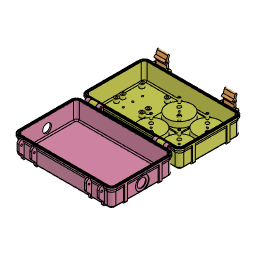
Rugged Relay Box Parametric_Microchallenge 03_MDEF v3 (Autodesk Fusion 360 design; units mm, degrees)
Autodesk Fusion 360 part; units mm, degrees
note: some values were not read from the file. Set by a fixed rule: which face or edge a step refers to.
(part 1 of 2)
sketch "Sketch1" plane through (0, 0, 0) normal (0, 1, 0) x (1, 0, 0) in component "Box"
  line L0 (45, -78) -> (-45, -78)
  line L1 (-48, -75) -> (-48, 75)
  line L2 (-45, 78) -> (45, 78)
  line L3 (48, 75) -> (48, -75)
  line L4 (48, -78) -> (-48, 78) construction
  line L5 (-48, -78) -> (48, 78) construction
  arc A0 (-45, 78) -> (-48, 75) centre (-45, 75) ccw
  arc A1 (48, 75) -> (45, 78) centre (45, 75) ccw
  arc A2 (45, -78) -> (48, -75) centre (45, -75) ccw
  arc A3 (-48, -75) -> (-45, -78) centre (-45, -75) ccw
  dimension "d6" = 156
  dimension "d7" = 96
  dimension "d9" = 3
  constraint horizontal L0
  constraint perpendicular L0 L1
  constraint parallel L0 L2
  constraint parallel L1 L3
  constraint coincident L4 origin
  constraint coincident L5 origin
  constraint coincident L4.end L2
  constraint coincident L4.end L1
  constraint tangent L2 A0
  constraint tangent L1 A0
  constraint coincident L5.end L2
  constraint coincident L5.end L3
  constraint tangent L2 A1
  constraint tangent L3 A1
  constraint coincident L4.start L3
  constraint coincident L4.start L0
  constraint tangent L3 A2
  constraint tangent L0 A2
  constraint coincident L5.start L0
  constraint coincident L5.start L1
  constraint tangent L0 A3
  constraint tangent L1 A3
  constraint equal A0 A1
  constraint equal A0 A3
  constraint equal A2 A3
  measures "d6" distance of L0 L2
  measures "d7" distance of L1 L3
  measures "d9" radius of A1
sketch "Sketch2" plane through (0, 0, 0) normal (0, 0, 1) x (1, 0, 0) in component "Box"
  line L0 (0, 0) -> (48, 0)
  line L1 (48, 0) -> (48, 2.4)
  line L2 (50, 4.4) -> (50, 32.4)
  line L3 (50, 32.4) -> (51.23, 32.4)
  line L4 (51.23, 32.4) -> (51.23, 30.4)
  line L5 (51.23, 30.4) -> (53.03, 30.4)
  line L6 (53.03, 30.4) -> (53.03, 32.4)
  line L7 (53.03, 32.4) -> (54.26, 32.4)
  line L8 (54.26, 32.4) -> (54.26, 29.4)
  line L9 (58.1865, 0) -> (48, 0)
  line L10 (54.26, 29.4) -> (52.4, 29.4)
  line L11 (52.4, 29.4) -> (52.4, 25)
  line L12 (52.4, 25) -> (52.4, 3.4059)
  line L13 (52.4, 25) -> (54.26, 29.4)
  line L14 (50, 4.4) -> (48, 2.4)
  line L15 (48.9941, 0) -> (52.4, 3.4059)
  line L16 (58.1865, 0) -> (61.26, 3.0735)
  line L17 (54.26, 32.4) -> (56.26, 32.4)
  line L18 (61.26, 27.4) -> (61.26, 3.0735)
  arc A0 (61.26, 27.4) -> (56.26, 32.4) centre (56.26, 27.4) ccw
  circle A1 centre (56.76, 24.4) radius 1.7
  line L19 (0, 0) -> (0, 60)
  line L20 (-61.26, 27.4) -> (-61.26, 3.0735)
  line L21 (-51.23, 32.4) -> (-51.23, 30.4)
  line L22 (-52.4, 25) -> (-54.26, 29.4)
  line L23 (-50, 4.4) -> (-50, 32.4)
  line L24 (-48, 0) -> (-48, 2.4)
  line L25 (-51.23, 30.4) -> (-53.03, 30.4)
  line L26 (-48.9941, 0) -> (-52.4, 3.4059)
  line L27 (-52.4, 25) -> (-52.4, 3.4059)
  line L28 (-50, 4.4) -> (-48, 2.4)
  line L29 (-54.26, 32.4) -> (-54.26, 29.4)
  line L30 (-58.1865, 0) -> (-61.26, 3.0735)
  line L31 (-52.4, 29.4) -> (-52.4, 25)
  line L32 (-53.03, 32.4) -> (-54.26, 32.4)
  line L33 (-53.03, 30.4) -> (-53.03, 32.4)
  line L34 (-58.1865, 0) -> (-48, 0)
  line L35 (-54.26, 29.4) -> (-52.4, 29.4)
  line L36 (-50, 32.4) -> (-51.23, 32.4)
  line L37 (52.4, 29.4) -> (50, 29.4)
  line L38 (-52.4, 29.4) -> (-50, 29.4)
  circle A2 centre (-57.86, 32.4) radius 1.7
  circle A3 centre (-57.86, 32.4) radius 3.4
  line L39 (-61.26, 32.4) -> (-61.26, 27.4)
  line L40 (-54.26, 32.4) -> (-54.46, 32.4)
  line L41 (-60.2642, 29.9958) -> (-50, 19.7317)
  line L42 (-60.2642, 29.9958) -> (-39.091, 29.9958) construction
  line L43 (-57.86, 32.4) -> (-54.26, 32.4)
  line L44 (51.6245, 0) -> (54.26, 2.6355)
  line L45 (54.26, 2.6355) -> (54.26, 8.4)
  line L46 (54.26, 8.4) -> (61.26, 15.4)
  line L47 (-51.6245, 0) -> (-54.26, 2.6355)
  line L48 (-54.26, 2.6355) -> (-54.26, 20.4)
  line L49 (-54.26, 20.4) -> (-61.26, 27.4)
  point P0 (61.26, 32.4)
  point P1 (-61.26, 32.4)
  dimension "d12" = 48
  dimension "d13" = 2.4
  dimension "d15" = 1.23
  dimension "d16" = 2
  dimension "d17" = 1.8
  dimension "d18" = 2
  dimension "d20" = 3
  dimension "d23" = 4.4
  dimension "d26" = 2.4
  dimension "d27" = 2
  dimension "d28" = 2
  dimension "d29" = 32.4
  dimension "d30" = 6.5
  dimension "d61" = 7
  dimension "d62" = 5
  dimension "d63" = 3.4
  dimension "d64" = 8
  dimension "d65" = 4.5
  dimension "d129" = 1.23
  dimension "d131" = 2.4
  dimension "d137" = 3.4
  dimension "d138" = 3.6
  dimension "d139" = 6.8
  dimension "d140" = 45
  dimension "d111" = 1.86
  dimension "d113" = 1.86
  dimension "d114" = 17
  dimension "d123" = 5
  constraint coincident L0.start L19.start
  constraint horizontal L0
  constraint perpendicular L0 L1
  constraint perpendicular L2 L3
  constraint perpendicular L3 L4
  constraint perpendicular L4 L5
  constraint perpendicular L5 L6
  constraint perpendicular L6 L7
  constraint perpendicular L7 L8
  constraint perpendicular L1 L9
  constraint perpendicular L8 L10
  constraint perpendicular L10 L11
  constraint perpendicular L9 L12
  constraint coincident L9 L15.start
  constraint vertical L2
  constraint perpendicular L8 L17
  constraint perpendicular L7 L18
  constraint coincident P0 L17
  constraint coincident P0 L18
  constraint tangent L17 A0
  constraint tangent L18 A0
  constraint perpendicular L0 L19
  constraint symmetric L0.end L19 L24.start
  constraint symmetric L1.end L19 L24.end
  constraint symmetric L2.end L19 L23.end
  constraint symmetric L3.end L19 L21.start
  constraint symmetric L4.end L19 L21.end
  constraint symmetric L5.end L19 L25.end
  constraint symmetric L6.end L19 L32.start
  constraint symmetric L7.end L19 L29.start
  constraint symmetric L8.end L19 L22.end
  constraint symmetric L10.end L19 L31.start
  constraint symmetric L11.end L19 L22.start
  constraint symmetric L2.start L19 L23.start
  constraint symmetric L15.start L19 L26.start
  constraint symmetric L12.end L19 L26.end
  constraint symmetric L9.start L19 L30.start
  constraint symmetric P0 L19 P1
  constraint symmetric L16.end L19 L20.end
  constraint symmetric L18.start L19 L20.start
  constraint coincident L2 L37.end
  constraint perpendicular L2 L37
  constraint coincident L23 L38.end
  constraint perpendicular L23 L38
  constraint concentric A2 A3
  constraint coincident P1 L39.start
  constraint coincident A3 L40.end
  constraint horizontal L42
  constraint coincident A3 L41.start
  constraint tangent A3 L41
  constraint coincident L23 L41.end
  constraint coincident A2.centre A3.centre
  constraint perpendicular L29 L43
  constraint horizontal L40
  constraint coincident L9 L44.start
  constraint perpendicular L9 L45
  constraint coincident L18 L46.end
  constraint collinear L8 L45
  constraint parallel L15 L44
  constraint symmetric L19 L44.start L47.start
  constraint symmetric L19 L44.end L47.end
  constraint parallel L44 L46
  constraint parallel L27 L48
  constraint coincident L20 L39.end
  constraint parallel L47 L49
  measures "d12" distance of L0.start L0.end
  measures "d13" distance of L0.end L1.end
  measures "d15" distance of L2.end L3.end
  measures "d16" distance of L3.end L4.end
  measures "d17" distance of L4.end L5.end
  measures "d18" distance of L5.end L6.end
  measures "d20" distance of L7.end L8.end
  measures "d23" distance of L10.end L11.end
  measures "d26" distance of L14 L15
  measures "d27" vertical distance of L1.end L2.start
  measures "d28" horizontal distance of L1.end L2.start
  measures "d29" distance of L0.end L7
  measures "d30" distance of L15 L16
  measures "d61" distance of L7.end P0
  measures "d62" radius of A0
  measures "d63" diameter of A1
  measures "d64" distance of L17 A1.centre
  measures "d65" distance of L18 A1.centre
  measures "d129" distance of L6 L8
  measures "d131" distance of L2 L12
  measures "d137" diameter of A2
  measures "d138" distance of L29.start A2.centre
  measures "d139" diameter of A3
  measures "d140" angle of L41 L42
  measures "d111" distance of L15 L44
  measures "d113" distance of L8 L11
  measures "d114" distance of L17 L46.end
  measures "d123" distance of L43 L20.start
extrude "Extrude1" add sketch "Sketch1" along normal blind 2.4 makes body 1 in component "Box"
sweep "Sweep1" add profiles "Sketch2" path "Sketch1" along A2 L0 A3 L1 A0 L2 A1 L3 section 1 contours L1 L2 L9 L11 L12 L14 L15 L37 | L2 L3 L4 L5 L6 L7 L8 L10 L37 | L10 L11 L13 bodies 1 in component "Box"
ref_plane "WorkPlane2" through (-32, 0, 0) normal (1, 0, 0) x (0, 1, 0) in component "Box"
sketch "Sketch4" plane through (-32, 0, 0) normal (1, 0, 0) x (0, 0, -1) in component "Box"
  line L0 (0, 0) -> (-78, 0)
  line L1 (-78, 0) -> (-78, 2.4)
  line L2 (-78, 2.4) -> (-80, 2.4)
  line L3 (-80, 2.4) -> (-80, 4.4)
  line L4 (-80, 4.4) -> (-78, 2.4)
  line L5 (-80, 2.4) -> (-80, 5)
  line L6 (-80, 2.4) -> (-80, 29.4)
  line L7 (-80, 29.4) -> (-84.26, 29.4)
  line L8 (-84.26, 29.4) -> (-84.26, 2.6355)
  line L9 (-81.6245, 0) -> (-78, 0)
  line L10 (-81.6245, 0) -> (-84.26, 2.6355)
  line L11 (0, 0) -> (0, 70)
  line L12 (81.6245, 0) -> (84.26, 2.6355)
  line L13 (81.6245, 0) -> (78, 0)
  line L14 (80, 2.4) -> (80, 5)
  line L15 (80, 2.4) -> (80, 29.4)
  line L16 (80, 4.4) -> (78, 2.4)
  line L17 (80, 2.4) -> (80, 4.4)
  line L18 (80, 29.4) -> (84.26, 29.4)
  line L19 (84.26, 29.4) -> (84.26, 2.6355)
  line L20 (78, 0) -> (78, 2.4)
  line L21 (78, 2.4) -> (80, 2.4)
  dimension "d47" = 78
  dimension "d48" = 2.4
  dimension "d49" = 2
  dimension "d50" = 2
  dimension "d52" = 4.26
  dimension "d53" = 4.26
  dimension "d56" = 29.4
  constraint coincident L0.start L11.start
  constraint horizontal L0
  constraint perpendicular L0 L1
  constraint perpendicular L1 L2
  constraint perpendicular L2 L3
  constraint coincident L3 L5.end
  constraint perpendicular L2 L6
  constraint perpendicular L6 L7
  constraint perpendicular L7 L8
  constraint perpendicular L1 L9
  constraint perpendicular L0 L11
  constraint symmetric L0.end L11 L13.end
  constraint symmetric L1.end L11 L16.end
  constraint symmetric L2.end L11 L14.start
  constraint symmetric L3.end L11 L16.start
  constraint symmetric L5.end L11 L14.end
  constraint symmetric L6.end L11 L15.end
  constraint symmetric L7.end L11 L18.end
  constraint symmetric L8.end L11 L12.end
  constraint symmetric L9.start L11 L12.start
  measures "d47" distance of L0.start L0.end
  measures "d48" distance of L0.end L1.end
  measures "d49" distance of L1.end L2.end
  measures "d50" distance of L2.end L3.end
  measures "d52" distance of L6.end L7.end
  measures "d53" distance of L4 L10
  measures "d56" distance of L7 L9
extrude "Extrude2" add sketch "Sketch4" along normal blind 5 bodies 1 in component "Box"
ref_plane "WorkPlane3" through (32, 0, 0) normal (1, 0, 0) x (0, 1, 0) in component "Box"
sketch "Sketch5" plane through (32, 0, 0) normal (1, 0, 0) x (0, 0, -1) in component "Box"
  line L0 (-80, 2.4) -> (-80, 29.4)
  line L1 (-80, 4.4) -> (-78, 2.4)
  line L2 (-78, 2.4) -> (-80, 2.4)
  line L3 (-78, 0) -> (-78, 2.4)
  line L4 (-81.6245, 0) -> (-78, 0)
  line L5 (-81.6245, 0) -> (-84.26, 2.6355)
  line L6 (-84.26, 29.4) -> (-84.26, 2.6355)
  line L7 (-80, 29.4) -> (-84.26, 29.4)
  line L8 (80, 29.4) -> (84.26, 29.4)
  line L9 (84.26, 29.4) -> (84.26, 2.6355)
  line L10 (80, 2.4) -> (80, 29.4)
  line L11 (80, 4.4) -> (78, 2.4)
  line L12 (78, 2.4) -> (80, 2.4)
  line L13 (81.6245, 0) -> (84.26, 2.6355)
  line L14 (78, 0) -> (78, 2.4)
  line L15 (81.6245, 0) -> (78, 0)
extrude "Extrude3" add sketch "Sketch5" against normal blind 5 bodies 1 in component "Box"
ref_plane "WorkPlane4" through (0, 0, -70) normal (0, 0, 1) x (1, 0, 0) in component "Box"
sketch "Sketch6" plane through (0, 0, -70) normal (0, 0, 1) x (1, 0, 0) in component "Box"
  line L0 (54.26, 32.4) -> (56.26, 32.4)
  line L1 (61.26, 27.4) -> (61.26, 3.0735)
  arc A0 (61.26, 27.4) -> (56.26, 32.4) centre (56.26, 27.4) ccw
  line L2 (58.1865, 0) -> (61.26, 3.0735)
  line L3 (58.1865, 0) -> (48, 0)
  line L4 (48, 0) -> (48, 2.4)
  line L5 (50, 4.4) -> (48, 2.4)
  line L6 (50, 4.4) -> (50, 32.4)
  line L7 (52.4, 29.4) -> (50, 29.4)
  line L8 (54.26, 29.4) -> (52.4, 29.4)
  line L9 (54.26, 32.4) -> (54.26, 29.4)
  line L10 (-50, 4.4) -> (-50, 32.4)
  line L11 (-52.4, 29.4) -> (-50, 29.4)
  line L12 (-54.26, 29.4) -> (-52.4, 29.4)
  line L13 (-54.26, 32.4) -> (-54.26, 29.4)
  line L14 (-61.26, 27.4) -> (-61.26, 3.0735)
  line L15 (-58.1865, 0) -> (-61.26, 3.0735)
  line L16 (-58.1865, 0) -> (-48, 0)
  line L17 (-48, 0) -> (-48, 2.4)
  line L18 (-50, 4.4) -> (-48, 2.4)
  circle A1 centre (56.76, 24.4) radius 1.7
  line L19 (-61.26, 32.4) -> (-61.26, 27.4)
  circle A2 centre (-57.86, 32.4) radius 3.4
  circle A3 centre (-57.86, 32.4) radius 1.7
  line L20 (-54.26, 32.4) -> (-54.46, 32.4)
  line L21 (-60.2642, 29.9958) -> (-50, 19.7317)
  line L22 (54.26, 8.4) -> (61.26, 15.4)
  line L23 (54.26, 2.6355) -> (54.26, 8.4)
  line L24 (51.6245, 0) -> (54.26, 2.6355)
  line L25 (-51.6245, 0) -> (-54.26, 2.6355)
  line L26 (-54.26, 2.6355) -> (-54.26, 20.4)
  line L27 (-54.26, 20.4) -> (-61.26, 27.4)
  point P0 (61.26, 32.4)
  point P1 (56.76, 24.4)
extrude "Extrude10" add sketch "Sketch6" along normal blind 3.2 contours L0 L1 A0 L3 L4 L5 L6 L7 L8 L9 L22 L23 L24 | L10 L16 L17 L18 L19 A2 L21 L25 L26 L27 | L10 L11 L12 L13 A2 L20 L21 | A2 bodies 1 in component "Box"
extrude "Extrude17" add sketch "Sketch6" along normal blind 6.2 contours L10 L11 L12 L13 A2 L20 L21 | A2 bodies 1 in component "Box"
ref_plane "WorkPlane5" through (0, 0, -45) normal (0, 0, 1) x (1, 0, 0) in component "Box"
sketch "Sketch7" plane through (0, 0, -45) normal (0, 0, 1) x (1, 0, 0) in component "Box"
  line L0 (-48, 0) -> (-48, 2.4)
  line L1 (-50, 4.4) -> (-48, 2.4)
  line L2 (-50, 4.4) -> (-50, 32.4)
  line L3 (-52.4, 29.4) -> (-50, 29.4)
  line L4 (-54.26, 29.4) -> (-52.4, 29.4)
  line L5 (-54.26, 32.4) -> (-54.26, 29.4)
  line L6 (-61.26, 27.4) -> (-61.26, 3.0735)
  line L7 (-58.1865, 0) -> (-61.26, 3.0735)
  line L8 (-58.1865, 0) -> (-48, 0)
  line L9 (48, 0) -> (48, 2.4)
  line L10 (50, 4.4) -> (48, 2.4)
  line L11 (50, 4.4) -> (50, 32.4)
  line L12 (52.4, 29.4) -> (50, 29.4)
  line L13 (54.26, 29.4) -> (52.4, 29.4)
  line L14 (54.26, 32.4) -> (54.26, 29.4)
  line L15 (54.26, 32.4) -> (56.26, 32.4)
  arc A0 (61.26, 27.4) -> (56.26, 32.4) centre (56.26, 27.4) ccw
  line L16 (61.26, 27.4) -> (61.26, 3.0735)
  line L17 (58.1865, 0) -> (61.26, 3.0735)
  line L18 (58.1865, 0) -> (48, 0)
  circle A1 centre (56.76, 24.4) radius 1.7 construction
  line L19 (-61.26, 32.4) -> (-61.26, 27.4)
  circle A2 centre (-57.86, 32.4) radius 3.4
  line L20 (-54.26, 32.4) -> (-54.46, 32.4)
  circle A3 centre (-57.86, 32.4) radius 1.7 construction
  line L21 (-60.2642, 29.9958) -> (-50, 19.7317)
  circle A4 centre (56.76, 24.4) radius 1.425
  circle A5 centre (-57.86, 32.4) radius 1.425
  line L22 (-51.6245, 0) -> (-54.26, 2.6355)
  line L23 (54.26, 8.4) -> (61.26, 15.4)
  line L24 (54.26, 2.6355) -> (54.26, 8.4)
  line L25 (51.6245, 0) -> (54.26, 2.6355)
  line L26 (-54.26, 2.6355) -> (-54.26, 20.4)
  line L27 (-54.26, 20.4) -> (-61.26, 27.4)
  dimension "d24" = 2.85
  dimension "d25" = 2.85
  constraint concentric A1 A4
  constraint concentric A2 A5
  measures "d24" diameter of A4
  measures "d25" diameter of A5
extrude "Extrude11" add sketch "Sketch7" against normal blind 3.2 contours L0 L1 L2 L8 L19 A2 L21 L22 L26 L27 | L2 L3 L4 L5 A2 L20 L21 | A2 | L9 L10 L11 L12 L13 L14 L15 A0 L16 L18 L23 L24 L25 bodies 1 in component "Box"
extrude "Extrude18" add sketch "Sketch7" against normal blind 6.2 contours L2 L3 L4 L5 A2 L20 L21 | A2 bodies 1 in component "Box"
ref_plane "WorkPlane6" through (0, 0, 70) normal (0, 0, 1) x (1, 0, 0) in component "Box"
sketch "Sketch8" plane through (0, 0, 70) normal (0, 0, 1) x (1, 0, 0) in component "Box"
  line L0 (-61.26, 27.4) -> (-61.26, 3.0735)
  line L1 (-54.26, 32.4) -> (-54.26, 29.4)
  line L2 (-54.26, 29.4) -> (-52.4, 29.4)
  line L3 (-52.4, 29.4) -> (-50, 29.4)
  line L4 (-50, 4.4) -> (-50, 32.4)
  line L5 (-50, 4.4) -> (-48, 2.4)
  line L6 (-48, 0) -> (-48, 2.4)
  line L7 (-58.1865, 0) -> (-48, 0)
  line L8 (-58.1865, 0) -> (-61.26, 3.0735)
  line L9 (48, 0) -> (48, 2.4)
  line L10 (50, 4.4) -> (48, 2.4)
  line L11 (50, 4.4) -> (50, 32.4)
  line L12 (52.4, 29.4) -> (50, 29.4)
  line L13 (54.26, 29.4) -> (52.4, 29.4)
  line L14 (54.26, 32.4) -> (54.26, 29.4)
  line L15 (54.26, 32.4) -> (56.26, 32.4)
  arc A0 (61.26, 27.4) -> (56.26, 32.4) centre (56.26, 27.4) ccw
  line L16 (61.26, 27.4) -> (61.26, 3.0735)
  line L17 (58.1865, 0) -> (61.26, 3.0735)
  circle A1 centre (56.76, 24.4) radius 1.7
  line L18 (58.1865, 0) -> (48, 0)
  line L19 (-61.26, 32.4) -> (-61.26, 27.4)
  circle A2 centre (-57.86, 32.4) radius 3.4
  circle A3 centre (-57.86, 32.4) radius 1.7
  line L20 (-54.26, 32.4) -> (-54.46, 32.4)
  line L21 (-60.2642, 29.9958) -> (-50, 19.7317)
  line L22 (54.26, 8.4) -> (61.26, 15.4)
  line L23 (54.26, 2.6355) -> (54.26, 8.4)
  line L24 (51.6245, 0) -> (54.26, 2.6355)
  line L25 (-51.6245, 0) -> (-54.26, 2.6355)
  line L26 (-54.26, 2.6355) -> (-54.26, 20.4)
  line L27 (-54.26, 20.4) -> (-61.26, 27.4)
extrude "Extrude12" add sketch "Sketch8" against normal blind 3.2 contours L4 L5 L6 L7 L19 A2 L21 L25 L26 L27 | A2 | L1 L2 L3 L4 A2 L20 L21 | L9 L10 L11 L12 L13 L14 L15 A0 L16 L18 L22 L23 L24 bodies 1 in component "Box"
extrude "Extrude19" add sketch "Sketch8" against normal blind 6.2 contours A2 | L1 L2 L3 L4 A2 L20 L21 bodies 1 in component "Box"
ref_plane "WorkPlane7" through (0, 0, 45) normal (0, 0, 1) x (1, 0, 0) in component "Box"
sketch "Sketch9" plane through (0, 0, 45) normal (0, 0, 1) x (1, 0, 0) in component "Box"
  line L0 (58.1865, 0) -> (61.26, 3.0735)
  line L1 (58.1865, 0) -> (48, 0)
  line L2 (61.26, 27.4) -> (61.26, 3.0735)
  arc A0 (61.26, 27.4) -> (56.26, 32.4) centre (56.26, 27.4) ccw
  line L3 (54.26, 32.4) -> (56.26, 32.4)
  line L4 (54.26, 32.4) -> (54.26, 29.4)
  line L5 (54.26, 29.4) -> (52.4, 29.4)
  line L6 (52.4, 29.4) -> (50, 29.4)
  line L7 (50, 4.4) -> (50, 32.4)
  line L8 (50, 4.4) -> (48, 2.4)
  line L9 (48, 0) -> (48, 2.4)
  line L10 (-48, 0) -> (-48, 2.4)
  line L11 (-50, 4.4) -> (-48, 2.4)
  line L12 (-50, 4.4) -> (-50, 32.4)
  line L13 (-52.4, 29.4) -> (-50, 29.4)
  line L14 (-54.26, 29.4) -> (-52.4, 29.4)
  line L15 (-54.26, 32.4) -> (-54.26, 29.4)
  line L16 (-61.26, 27.4) -> (-61.26, 3.0735)
  line L17 (-58.1865, 0) -> (-61.26, 3.0735)
  line L18 (-58.1865, 0) -> (-48, 0)
  circle A1 centre (56.76, 24.4) radius 1.7 construction
  line L19 (-61.26, 32.4) -> (-61.26, 27.4)
  circle A2 centre (-57.86, 32.4) radius 3.4
  circle A3 centre (-57.86, 32.4) radius 1.7 construction
  line L20 (-54.26, 32.4) -> (-54.46, 32.4)
  line L21 (-60.2642, 29.9958) -> (-50, 19.7317)
  circle A4 centre (56.76, 24.4) radius 1.425
  circle A5 centre (-57.86, 32.4) radius 1.425
  line L22 (54.26, 8.4) -> (61.26, 15.4)
  line L23 (54.26, 2.6355) -> (54.26, 8.4)
  line L24 (51.6245, 0) -> (54.26, 2.6355)
  line L25 (-51.6245, 0) -> (-54.26, 2.6355)
  line L26 (-54.26, 2.6355) -> (-54.26, 20.4)
  line L27 (-54.26, 20.4) -> (-61.26, 27.4)
  point P0 (56.26, 27.4)
  dimension "d39" = 2.85
  dimension "d40" = 2.85
  constraint concentric A1 A4
  constraint concentric A2 A5
  measures "d39" diameter of A4
  measures "d40" diameter of A5
extrude "Extrude13" add sketch "Sketch9" along normal blind 3.2 contours L1 L2 A0 L3 L4 L5 L6 L7 L8 L9 L22 L23 L24 | L10 L11 L12 L18 L19 A2 L21 L25 L26 L27 | L12 L13 L14 L15 A2 L20 L21 | A2 bodies 1 in component "Box"
extrude "Extrude20" add sketch "Sketch9" along normal blind 6.2 contours L12 L13 L14 L15 A2 L20 L21 | A2 bodies 1 in component "Box"
fillet "Fillet2" radius 1 40 edges at (-54.26, 2.6355, 68.4) (-54.26, 20.4, 68.4) (-54.26, 20.4, 46.6) (-54.26, 2.6355, 46.6) (-54.26, 2.6355, -46.6) (-54.26, 20.4, -46.6) (-54.26, 20.4, -68.4) (-54.26, 2.6355, -68.4) (-29.5, 2.6355, 84.26) (29.5, 2.6355, 84.26) (54.26, 2.6355, 68.4) (54.26, 8.4, 68.4) (54.26, 2.6355, 46.6) (54.26, 8.4, 46.6) (54.26, 8.4, -46.6) (54.26, 2.6355, -46.6) (54.26, 2.6355, -68.4) (54.26, 8.4, -68.4) (29.5, 2.6355, -84.26) (-29.5, 2.6355, -84.26) (52.4, 3.4059, 72.5) (50.2326, 3.4059, 80.2326) (38.5, 3.4059, 82.4) (0, 3.4059, 82.4) (-38.5, 3.4059, 82.4) (-50.2326, 3.4059, 80.2326) (-52.4, 3.4059, 72.5) (52.4, 3.4059, 57.5) (52.4, 3.4059, 0) (52.4, 3.4059, -57.5) (38.5, 3.4059, -82.4) (50.2326, 3.4059, -80.2326) (52.4, 3.4059, -72.5) (0, 3.4059, -82.4) (-52.4, 3.4059, -72.5) (-50.2326, 3.4059, -80.2326) (-38.5, 3.4059, -82.4) (-52.4, 3.4059, -57.5) (-52.4, 3.4059, 0) (-52.4, 3.4059, 57.5) 17 faces at (-50.7477, 0, 46.0667) (-50.7477, 0, 68.9333) (-50.7477, 0, -46.0667) (-49.8709, 0, -67.8667) (50.7477, 0, -68.9333) (50.7477, 0, -46.0667) (50.7477, 0, 46.0667) (50.7477, 0, 68.9333) (-48.3314, 0, -22.2667) (30.3333, 0, -79.8709) (-28.6667, 0, -79.8709) (48.3314, 0, 22.2667) (28.6667, 0, 79.8709) (-30.3333, 0, 79.8709) (16, 0, 25) (10.6667, 0, -78.3314) (10.6667, 0, 78.3314) on bodies 1 in component "Box"
fillet "Fillet3" radius 3 8 edges at (61.26, 15.4, 68.4) (61.26, 15.4, 46.6) (61.26, 15.4, -46.6) (61.26, 15.4, -68.4) (-61.26, 27.4, -68.4) (-61.26, 27.4, -46.6) (-61.26, 27.4, 46.6) (-61.26, 27.4, 68.4) on bodies 1 in component "Box"
copy_body "Body->Comp1" bodies 1 removing the originals makes body 2 in component "Box (1)"
sketch "Sketch10" plane through (0, 0, 0) normal (0, 0, 1) x (1, 0, 0) in component "Box"
  circle A0 centre (152.4867, 44.0068) radius 1.6
  circle A1 centre (152.4867, 44.0068) radius 4
  circle A2 centre (152.4867, 60.0068) radius 1.6
  circle A3 centre (152.4867, 60.0068) radius 4
  arc A4 (152.4867, 60.0068) -> (152.4867, 44.0068) centre (171.1154, 52.0068) ccw
  arc A5 (151.0165, 60.6382) -> (151.0165, 43.3755) centre (171.1154, 52.0068) ccw
  arc A6 (153.9568, 59.3755) -> (153.9568, 44.6382) centre (171.1154, 52.0068) ccw
  line L0 (153.4854, 42.7568) -> (156.2863, 42.7568)
  line L1 (152.4867, 44.0068) -> (149.3136, 34.5236)
  circle A7 centre (149.3136, 34.5236) radius 1.6
  line L2 (150.9693, 44.5145) -> (147.7963, 35.0313)
  line L3 (154.004, 43.4992) -> (150.8309, 34.0159)
  line L4 (152.4973, 45.6068) -> (152.8792, 47.9875)
  line L5 (152.4867, 60.0068) -> (152.4867, 44.0068) construction
  dimension "d98" = 3.2
  dimension "d99" = 8
  dimension "d100" = 16
  dimension "d101" = 3.2
  dimension "d102" = 8
  dimension "d105" = 3.2
  dimension "d66" = 10
  dimension "d67" = 161.5
  dimension "d69" = 1.25
  constraint concentric A0 A1
  constraint coincident A0.centre A1.centre
  constraint coincident A2.centre A3.centre
  constraint concentric A2 A3
  constraint coincident A0 L0.start
  constraint coincident A1 L0.end
  constraint coincident L1.end A7.centre
  constraint coincident A0 L4.start
  constraint coincident A6 L4.end
  constraint coincident A1 L4.end
  constraint concentric A4 A6
  constraint concentric A4 A5
  constraint vertical L5
  constraint coincident A2 A6.start
  constraint tangent A2 A6
  constraint tangent A2 A5
  constraint coincident A2 A5.start
  constraint coincident A0 A5.end
  constraint coincident A0 A6.end
  constraint parallel L1 L2
  constraint parallel L1 L3
  constraint coincident A0 L3.start
  constraint coincident A0 L2.start
  constraint tangent A0 L2
  constraint tangent A0 L3
  constraint coincident A7 L2.end
  constraint coincident A7 L3.end
  constraint horizontal L0
  measures "d98" diameter of A0
  measures "d99" diameter of A1
  measures "d100" distance of A0.centre A2.centre
  measures "d101" diameter of A2
  measures "d102" diameter of A3
  measures "d105" diameter of A7
  measures "d66" distance of A0.centre L1.end
  measures "d67" angle of L1 L5
  measures "d69" distance of A0.centre L0
extrude "Extrude15" add sketch "Sketch10" along normal blind 18.2 separate body contours A0 A1 A4 L4 | A1 A3 A4 A6 | A0 A1 L0 L1 L3 | A1 L0 L3 | A0 A1 A4 A5 L2 | A1 A3 A4 A5 | A2 A3 A5 A6 | A2 A3 A4 A6 | A0 A1 A5 L1 L2 | A1 L1 A7 L3 | A1 A5 L2 | A2 A3 A4 A5 | A1 L1 A7 L2 | A7 makes body 3 in component "Box"
copy_body "Body->Comp3" bodies 3 removing the originals makes body 4 in component "Box Latch"
sketch "Sketch1 (2)" plane through (0, 0, 0) normal (0, 1, 0) x (1, 0, 0) in component "Lid"
  line L0 (45, -78) -> (-45, -78)
  line L1 (-48, -75) -> (-48, 75)
  line L2 (-45, 78) -> (45, 78)
  line L3 (48, 75) -> (48, -75)
  line L4 (48, -78) -> (-48, 78) construction
  line L5 (-48, -78) -> (48, 78) construction
  arc A0 (-45, 78) -> (-48, 75) centre (-45, 75) ccw
  arc A1 (48, 75) -> (45, 78) centre (45, 75) ccw
  arc A2 (45, -78) -> (48, -75) centre (45, -75) ccw
  arc A3 (-48, -75) -> (-45, -78) centre (-45, -75) ccw
  dimension "d6_1" = 156
  dimension "d7_1" = 96
  dimension "d9_1" = 3
  constraint horizontal L0
  constraint perpendicular L0 L1
  constraint parallel L0 L2
  constraint parallel L1 L3
  constraint coincident L4 origin
  constraint coincident L5 origin
  constraint coincident L4.end L2
  constraint coincident L4.end L1
  constraint tangent L2 A0
  constraint tangent L1 A0
  constraint coincident L5.end L2
  constraint coincident L5.end L3
  constraint tangent L2 A1
  constraint tangent L3 A1
  constraint coincident L4.start L3
  constraint coincident L4.start L0
  constraint tangent L3 A2
  constraint tangent L0 A2
  constraint coincident L5.start L0
  constraint coincident L5.start L1
  constraint tangent L0 A3
  constraint tangent L1 A3
  constraint equal A0 A1
  constraint equal A0 A3
  constraint equal A2 A3
  measures "d6_1" distance of L0 L2
  measures "d7_1" distance of L1 L3
  measures "d9_1" radius of A1
sketch "Sketch2 (2)" plane through (0, 0, 0) normal (0, 0, 1) x (1, 0, 0) in component "Lid"
  line L0 (0, 0) -> (48, 0)
  line L1 (48, 0) -> (48, 2.4)
  line L2 (50, 4.4) -> (50, 32.4)
  line L3 (50, 32.4) -> (51.23, 32.4)
  line L4 (51.23, 32.4) -> (51.23, 30.4)
  line L5 (51.23, 30.4) -> (53.03, 30.4)
  line L6 (53.03, 30.4) -> (53.03, 32.4)
  line L7 (53.03, 32.4) -> (54.26, 32.4)
  line L8 (54.26, 32.4) -> (54.26, 29.4)
  line L9 (58.1865, 0) -> (48, 0)
  line L10 (54.26, 29.4) -> (52.4, 29.4)
  line L11 (52.4, 29.4) -> (52.4, 25)
  line L12 (52.4, 25) -> (52.4, 3.4059)
  line L13 (52.4, 25) -> (54.26, 29.4)
  line L14 (50, 4.4) -> (48, 2.4)
  line L15 (48.9941, 0) -> (52.4, 3.4059)
  line L16 (58.1865, 0) -> (61.26, 3.0735)
  line L17 (54.26, 32.4) -> (56.26, 32.4)
  line L18 (61.26, 27.4) -> (61.26, 3.0735)
  arc A0 (61.26, 27.4) -> (56.26, 32.4) centre (56.26, 27.4) ccw
  circle A1 centre (56.76, 24.4) radius 1.7
  line L19 (0, 0) -> (0, 60)
  line L20 (-51.23, 32.4) -> (-51.23, 30.4)
  line L21 (-52.4, 25) -> (-54.26, 29.4)
  line L22 (-50, 4.4) -> (-50, 32.4)
  line L23 (-48, 0) -> (-48, 2.4)
  line L24 (-51.23, 30.4) -> (-53.03, 30.4)
  line L25 (-48.9941, 0) -> (-52.4, 3.4059)
  line L26 (-52.4, 25) -> (-52.4, 3.4059)
  line L27 (-50, 4.4) -> (-48, 2.4)
  line L28 (-54.26, 32.4) -> (-54.26, 29.4)
  line L29 (-52.4, 29.4) -> (-52.4, 25)
  line L30 (-53.03, 32.4) -> (-54.26, 32.4)
  line L31 (-53.03, 30.4) -> (-53.03, 32.4)
  line L32 (-54.26, 29.4) -> (-52.4, 29.4)
  line L33 (-50, 32.4) -> (-51.23, 32.4)
  line L34 (52.4, 29.4) -> (50, 29.4)
  line L35 (-52.4, 29.4) -> (-50, 29.4)
  line L36 (51.23, 32.4) -> (53.03, 32.4)
  line L37 (52.13, 32.4) -> (52.13, 33.3)
  line L38 (52.13, 33.3) -> (52.33, 33.3)
  line L39 (52.33, 33.3) -> (52.33, 33.06)
  line L40 (52.13, 33.3) -> (51.93, 33.3)
  line L41 (51.93, 33.3) -> (51.93, 33.06)
  line L42 (51.38, 32.4) -> (51.38, 30.4)
  line L43 (52.88, 30.4) -> (52.88, 32.4)
  line L44 (51.38, 32.4) -> (52.13, 33.3)
  line L45 (52.13, 33.3) -> (52.88, 32.4)
  circle A2 centre (-57.86, 32.4) radius 1.7
  circle A3 centre (-57.86, 32.4) radius 3.4
  line L46 (-54.26, 32.4) -> (-54.46, 32.4)
  line L47 (-60.2642, 29.9958) -> (-52.4, 22.1317)
  line L48 (-60.2642, 29.9958) -> (-89.0433, 29.9958) construction
  line L49 (-48, 0) -> (-48.9941, 0)
  line L50 (-58.1865, 0) -> (-48, 0)
  line L51 (-58.1865, 0) -> (-61.26, 3.0735)
  line L52 (-61.26, 27.4) -> (-61.26, 3.0735)
  line L53 (-61.26, 27.4) -> (-61.26, 32.4)
  line L54 (-57.86, 32.4) -> (-54.26, 32.4)
  line L55 (51.6245, 0) -> (54.26, 2.6355)
  line L56 (54.26, 2.6355) -> (54.26, 15.4)
  line L57 (54.26, 15.4) -> (61.26, 22.4)
  line L58 (-51.6245, 0) -> (-54.26, 2.6355)
  line L59 (-54.26, 2.6355) -> (-54.26, 20.4)
  line L60 (-54.26, 20.4) -> (-61.26, 27.4)
  point P0 (61.26, 32.4)
  point P1 (-61.26, 32.4)
  dimension "d12_1" = 48
  dimension "d13_1" = 2.4
  dimension "d15_1" = 1.23
  dimension "d16_1" = 2
  dimension "d17_1" = 1.8
  dimension "d18_1" = 2
  dimension "d19" = 1.23
  dimension "d20_1" = 3
  dimension "d23_1" = 4.4
  dimension "d26_1" = 2.4
  dimension "d27_1" = 2
  dimension "d28_1" = 2
  dimension "d29_1" = 32.4
  dimension "d30_1" = 6.5
  dimension "d61_1" = 7
  dimension "d62_1" = 5
  dimension "d63_1" = 3.4
  dimension "d64_1" = 8
  dimension "d65_1" = 4.5
  dimension "d134" = 2.4
  dimension "d135" = 0.15
  dimension "d136" = 0.15
  dimension "d137_1" = 79.611
  dimension "d138_1" = 0.24
  dimension "d139_1" = 0.24
  dimension "d156" = 3.4
  dimension "d157" = 3.6
  dimension "d158" = 6.8
  dimension "d159" = 45
  dimension "d116" = 1.86
  dimension "d117" = 1.86
  dimension "d118" = 10
  dimension "d125" = 5
  constraint coincident L0.start L19.start
  constraint horizontal L0
  constraint perpendicular L0 L1
  constraint perpendicular L2 L3
  constraint perpendicular L3 L4
  constraint perpendicular L4 L5
  constraint perpendicular L5 L6
  constraint perpendicular L6 L7
  constraint perpendicular L7 L8
  constraint perpendicular L1 L9
  constraint perpendicular L8 L10
  constraint perpendicular L10 L11
  constraint perpendicular L9 L12
  constraint coincident L9 L15.start
  constraint vertical L2
  constraint perpendicular L8 L17
  constraint perpendicular L7 L18
  constraint coincident P0 L17
  constraint coincident P0 L18
  constraint tangent L17 A0
  constraint tangent L18 A0
  constraint perpendicular L0 L19
  constraint symmetric L0.end L19 L23.start
  constraint symmetric L1.end L19 L23.end
  constraint symmetric L2.end L19 L22.end
  constraint symmetric L3.end L19 L20.start
  constraint symmetric L4.end L19 L20.end
  constraint symmetric L5.end L19 L24.end
  constraint symmetric L6.end L19 L30.start
  constraint symmetric L7.end L19 L28.start
  constraint symmetric L8.end L19 L21.end
  constraint symmetric L10.end L19 L29.start
  constraint symmetric L11.end L19 L21.start
  constraint symmetric L2.start L19 L22.start
  constraint symmetric L15.start L19 L25.start
  constraint symmetric L12.end L19 L25.end
  constraint symmetric P0 L19 P1
  constraint coincident L2 L34.end
  constraint perpendicular L2 L34
  constraint coincident L22 L35.end
  constraint perpendicular L22 L35
  constraint midpoint L36 L37.start
  constraint perpendicular L36 L37
  constraint perpendicular L37 L38
  constraint perpendicular L36 L39
  constraint perpendicular L39 L40
  constraint perpendicular L40 L41
  constraint coincident L36 L42.start
  constraint coincident L5 L42.end
  constraint perpendicular L5 L42
  constraint coincident L5 L43.start
  constraint coincident L36 L43.end
  constraint perpendicular L36 L43
  constraint coincident L44 L41.end
  constraint coincident L45 L39.end
  constraint concentric A2 A3
  constraint coincident A3 L46.end
  constraint horizontal L48
  constraint coincident A3 L47.start
  constraint coincident L26 L47.end
  constraint tangent A3 L47
  constraint symmetric L9.start L19 L50.start
  constraint symmetric L16.end L19 L51.end
  constraint symmetric L18.start L19 L52.start
  constraint coincident P1 L53.end
  constraint horizontal L46
  constraint coincident A2.centre A3.centre
  constraint perpendicular L28 L54
  constraint coincident L9 L55.start
  constraint perpendicular L9 L56
  constraint coincident L18 L57.end
  constraint parallel L55 L57
  constraint parallel L15 L55
  constraint collinear L8 L56
  constraint symmetric L19 L55.start L58.start
  constraint symmetric L19 L55.end L58.end
  constraint vertical L59
  constraint coincident L52 L53.start
  constraint parallel L58 L60
  measures "d12_1" distance of L0.start L0.end
  measures "d13_1" distance of L0.end L1.end
  measures "d15_1" distance of L2.end L3.end
  measures "d16_1" distance of L3.end L4.end
  measures "d17_1" distance of L4.end L5.end
  measures "d18_1" distance of L5.end L6.end
  measures "d19" distance of L6.end L7.end
  measures "d20_1" distance of L7.end L8.end
  measures "d23_1" distance of L10.end L11.end
  measures "d26_1" distance of L14 L15
  measures "d27_1" vertical distance of L1.end L2.start
  measures "d28_1" horizontal distance of L1.end L2.start
  measures "d29_1" distance of L0.end L7
  measures "d30_1" distance of L15 L16
  measures "d61_1" distance of L7.end P0
  measures "d62_1" radius of A0
  measures "d63_1" diameter of A1
  measures "d64_1" distance of L17 A1.centre
  measures "d65_1" distance of L18 A1.centre
  measures "d134" distance of L2 L12
  measures "d135" distance of L4 L42
  measures "d136" distance of L6 L43
  measures "d137_1" angle of L44 L45
  measures "d138_1" distance of L40.end L41.end
  measures "d139_1" distance of L38.end L39.end
  measures "d156" diameter of A2
  measures "d157" distance of L28.start A2.centre
  measures "d158" diameter of A3
  measures "d159" angle of L47 L48
  measures "d116" distance of L8 L11
  measures "d117" distance of L15 L55
  measures "d118" distance of L17 L57.end
  measures "d125" distance of L54 L52.start
extrude "Extrude1'" add sketch "Sketch1 (2)" along normal blind 2.4 separate body makes body 5 in component "Lid"
sweep "Sweep1'" add profiles "Sketch2 (2)" path "Sketch1 (2)" along A2 L0 A3 L1 A0 L2 A1 L3 section 1 contours L1 L2 L9 L11 L12 L14 L15 L34 | L2 L3 L4 L5 L6 L7 L8 L10 L34 | L10 L11 L13 | L4 L5 L36 L42 | L36 L37 L44 | L5 L36 L42 L43 | L5 L6 L36 L43 | L36 L37 L45 | L40 L41 L44 | L38 L39 L45 separate body makes body 6 in component "Lid"
ref_plane "WorkPlane2" through (-32, 0, 0) normal (1, 0, 0) x (0, 1, 0) in component "Lid"
sketch "Sketch4 (2)" plane through (-32, 0, 0) normal (1, 0, 0) x (0, 0, -1) in component "Lid"
  line L0 (0, 0) -> (-78, 0)
  line L1 (-78, 0) -> (-78, 2.4)
  line L2 (-78, 2.4) -> (-80, 2.4)
  line L3 (-80, 2.4) -> (-80, 4.4)
  line L4 (-80, 4.4) -> (-78, 2.4)
  line L5 (-80, 2.4) -> (-80, 5)
  line L6 (-80, 2.4) -> (-80, 29.4)
  line L7 (-80, 29.4) -> (-84.26, 29.4)
  line L8 (-84.26, 29.4) -> (-84.26, 2.6355)
  line L9 (-81.6245, 0) -> (-78, 0)
  line L10 (-81.6245, 0) -> (-84.26, 2.6355)
  line L11 (0, 0) -> (0, 70)
  line L12 (81.6245, 0) -> (84.26, 2.6355)
  line L13 (81.6245, 0) -> (78, 0)
  line L14 (80, 2.4) -> (80, 5)
  line L15 (80, 2.4) -> (80, 29.4)
  line L16 (80, 4.4) -> (78, 2.4)
  line L17 (80, 2.4) -> (80, 4.4)
  line L18 (80, 29.4) -> (84.26, 29.4)
  line L19 (84.26, 29.4) -> (84.26, 2.6355)
  line L20 (78, 0) -> (78, 2.4)
  line L21 (78, 2.4) -> (80, 2.4)
  dimension "d47_1" = 78
  dimension "d48_1" = 2.4
  dimension "d49_1" = 2
  dimension "d50_1" = 2
  dimension "d52_1" = 4.26
  dimension "d53_1" = 4.26
  dimension "d56_1" = 29.4
  constraint coincident L0.start L11.start
  constraint horizontal L0
  constraint perpendicular L0 L1
  constraint perpendicular L1 L2
  constraint perpendicular L2 L3
  constraint coincident L3 L5.end
  constraint perpendicular L2 L6
  constraint perpendicular L6 L7
  constraint perpendicular L7 L8
  constraint perpendicular L1 L9
  constraint perpendicular L0 L11
  constraint symmetric L0.end L11 L13.end
  constraint symmetric L1.end L11 L16.end
  constraint symmetric L2.end L11 L14.start
  constraint symmetric L3.end L11 L16.start
  constraint symmetric L5.end L11 L14.end
  constraint symmetric L6.end L11 L15.end
  constraint symmetric L7.end L11 L18.end
  constraint symmetric L8.end L11 L12.end
  constraint symmetric L9.start L11 L12.start
  measures "d47_1" distance of L0.start L0.end
  measures "d48_1" distance of L0.end L1.end
  measures "d49_1" distance of L1.end L2.end
  measures "d50_1" distance of L2.end L3.end
  measures "d52_1" distance of L6.end L7.end
  measures "d53_1" distance of L4 L10
  measures "d56_1" distance of L7 L9
extrude "Extrude2'" add sketch "Sketch4 (2)" along normal blind 5 bodies 6 5 in component "Lid"
ref_plane "WorkPlane3" through (32, 0, 0) normal (1, 0, 0) x (0, 1, 0) in component "Lid"
sketch "Sketch5 (2)" plane through (32, 0, 0) normal (1, 0, 0) x (0, 0, -1) in component "Lid"
  line L0 (-80, 2.4) -> (-80, 29.4)
  line L1 (-80, 4.4) -> (-78, 2.4)
  line L2 (-78, 2.4) -> (-80, 2.4)
  line L3 (-78, 0) -> (-78, 2.4)
  line L4 (-81.6245, 0) -> (-78, 0)
  line L5 (-81.6245, 0) -> (-84.26, 2.6355)
  line L6 (-84.26, 29.4) -> (-84.26, 2.6355)
  line L7 (-80, 29.4) -> (-84.26, 29.4)
  line L8 (80, 29.4) -> (84.26, 29.4)
  line L9 (84.26, 29.4) -> (84.26, 2.6355)
  line L10 (80, 2.4) -> (80, 29.4)
  line L11 (80, 4.4) -> (78, 2.4)
  line L12 (78, 2.4) -> (80, 2.4)
  line L13 (81.6245, 0) -> (84.26, 2.6355)
  line L14 (78, 0) -> (78, 2.4)
  line L15 (81.6245, 0) -> (78, 0)
extrude "Extrude3'" add sketch "Sketch5 (2)" against normal blind 5 bodies 6 in component "Lid"
ref_plane "WorkPlane4" through (0, 0, -70) normal (0, 0, 1) x (1, 0, 0) in component "Lid"
sketch "Sketch6 (2)" plane through (0, 0, -70) normal (0, 0, 1) x (1, 0, 0) in component "Lid"
  line L0 (54.26, 32.4) -> (56.26, 32.4)
  line L1 (61.26, 27.4) -> (61.26, 3.0735)
  arc A0 (61.26, 27.4) -> (56.26, 32.4) centre (56.26, 27.4) ccw
  line L2 (58.1865, 0) -> (61.26, 3.0735)
  line L3 (58.1865, 0) -> (48, 0)
  line L4 (48, 0) -> (48, 2.4)
  line L5 (50, 4.4) -> (48, 2.4)
  line L6 (50, 4.4) -> (50, 32.4)
  line L7 (52.4, 29.4) -> (50, 29.4)
  line L8 (54.26, 29.4) -> (52.4, 29.4)
  line L9 (54.26, 32.4) -> (54.26, 29.4)
  circle A1 centre (56.76, 24.4) radius 1.7
  line L10 (54.26, 15.4) -> (61.26, 22.4)
  line L11 (54.26, 2.6355) -> (54.26, 15.4)
  line L12 (51.6245, 0) -> (54.26, 2.6355)
  point P0 (61.26, 32.4)
  point P1 (56.76, 24.4)
extrude "Extrude10'" add sketch "Sketch6 (2)" along normal blind 3.2 contours L0 L1 A0 L3 L4 L5 L6 L7 L8 L9 L10 L11 L12 bodies 6 in component "Lid"
ref_plane "WorkPlane5" through (0, 0, -45) normal (0, 0, 1) x (1, 0, 0) in component "Lid"
sketch "Sketch7 (2)" plane through (0, 0, -45) normal (0, 0, 1) x (1, 0, 0) in component "Lid"
  line L0 (48, 0) -> (48, 2.4)
  line L1 (50, 4.4) -> (48, 2.4)
  line L2 (50, 4.4) -> (50, 32.4)
  line L3 (52.4, 29.4) -> (50, 29.4)
  line L4 (54.26, 29.4) -> (52.4, 29.4)
  line L5 (54.26, 32.4) -> (54.26, 29.4)
  line L6 (54.26, 32.4) -> (56.26, 32.4)
  arc A0 (61.26, 27.4) -> (56.26, 32.4) centre (56.26, 27.4) ccw
  line L7 (61.26, 27.4) -> (61.26, 3.0735)
  line L8 (58.1865, 0) -> (61.26, 3.0735)
  line L9 (58.1865, 0) -> (48, 0)
  circle A1 centre (56.76, 24.4) radius 1.7 construction
  circle A2 centre (56.76, 24.4) radius 1.425
  line L10 (54.26, 15.4) -> (61.26, 22.4)
  line L11 (54.26, 2.6355) -> (54.26, 15.4)
  line L12 (51.6245, 0) -> (54.26, 2.6355)
  dimension "d41" = 2.85
  constraint concentric A1 A2
  measures "d41" diameter of A2
extrude "Extrude11'" add sketch "Sketch7 (2)" against normal blind 3.2 contours L0 L1 L2 L3 L4 L5 L6 A0 L7 L9 L10 L11 L12 bodies 6 in component "Lid"
ref_plane "WorkPlane6" through (0, 0, 70) normal (0, 0, 1) x (1, 0, 0) in component "Lid"
sketch "Sketch8 (2)" plane through (0, 0, 70) normal (0, 0, 1) x (1, 0, 0) in component "Lid"
  line L0 (48, 0) -> (48, 2.4)
  line L1 (50, 4.4) -> (48, 2.4)
  line L2 (50, 4.4) -> (50, 32.4)
  line L3 (52.4, 29.4) -> (50, 29.4)
  line L4 (54.26, 29.4) -> (52.4, 29.4)
  line L5 (54.26, 32.4) -> (54.26, 29.4)
  line L6 (54.26, 32.4) -> (56.26, 32.4)
  arc A0 (61.26, 27.4) -> (56.26, 32.4) centre (56.26, 27.4) ccw
  line L7 (61.26, 27.4) -> (61.26, 3.0735)
  line L8 (58.1865, 0) -> (61.26, 3.0735)
  circle A1 centre (56.76, 24.4) radius 1.7
  line L9 (58.1865, 0) -> (48, 0)
  line L10 (54.26, 15.4) -> (61.26, 22.4)
  line L11 (54.26, 2.6355) -> (54.26, 15.4)
  line L12 (51.6245, 0) -> (54.26, 2.6355)
extrude "Extrude12'" add sketch "Sketch8 (2)" against normal blind 3.2 contours L0 L1 L2 L3 L4 L5 L6 A0 L7 L9 L10 L11 L12 bodies 6 in component "Lid"
ref_plane "WorkPlane7" through (0, 0, 45) normal (0, 0, 1) x (1, 0, 0) in component "Lid"
sketch "Sketch9 (2)" plane through (0, 0, 45) normal (0, 0, 1) x (1, 0, 0) in component "Lid"
  line L0 (58.1865, 0) -> (61.26, 3.0735)
  line L1 (58.1865, 0) -> (48, 0)
  line L2 (61.26, 27.4) -> (61.26, 3.0735)
  arc A0 (61.26, 27.4) -> (56.26, 32.4) centre (56.26, 27.4) ccw
  line L3 (54.26, 32.4) -> (56.26, 32.4)
  line L4 (54.26, 32.4) -> (54.26, 29.4)
  line L5 (54.26, 29.4) -> (52.4, 29.4)
  line L6 (52.4, 29.4) -> (50, 29.4)
  line L7 (50, 4.4) -> (50, 32.4)
  line L8 (50, 4.4) -> (48, 2.4)
  line L9 (48, 0) -> (48, 2.4)
  circle A1 centre (56.76, 24.4) radius 1.7 construction
  circle A2 centre (56.76, 24.4) radius 1.425
  line L10 (54.26, 15.4) -> (61.26, 22.4)
  line L11 (54.26, 2.6355) -> (54.26, 15.4)
  line L12 (51.6245, 0) -> (54.26, 2.6355)
  point P0 (56.26, 27.4)
  dimension "d42" = 2.85
  constraint concentric A1 A2
  measures "d42" diameter of A2
extrude "Extrude13'" add sketch "Sketch9 (2)" along normal blind 3.2 contours L1 L2 A0 L3 L4 L5 L6 L7 L8 L9 L10 L11 L12 bodies 6 in component "Lid"
ref_plane "WorkPlane8" through (0, 0, -57.5) normal (0, 0, 1) x (1, 0, 0) in component "Lid"
sketch "Sketch12" plane through (0, 0, -57.5) normal (0, 0, 1) x (1, 0, 0) in component "Lid"
  line L0 (-60.2642, 29.9958) -> (-52.4, 22.1317)
  circle A0 centre (-57.86, 32.4) radius 3.4
  circle A1 centre (-57.86, 32.4) radius 1.7
  line L1 (-54.26, 32.4) -> (-54.46, 32.4)
  line L2 (-54.26, 32.4) -> (-54.26, 29.4)
  line L3 (-52.4, 25) -> (-54.26, 29.4)
  line L4 (-52.4, 25) -> (-52.4, 3.4059)
  line L5 (-61.26, 27.4) -> (-61.26, 3.0735)
  line L6 (-61.26, 27.4) -> (-61.26, 32.4)
  line L7 (-58.1865, 0) -> (-61.26, 3.0735)
  line L8 (-58.1865, 0) -> (-48, 0)
  line L9 (-48.9941, 0) -> (-52.4, 3.4059)
  line L10 (-51.6245, 0) -> (-54.26, 2.6355)
  line L11 (-54.26, 20.4) -> (-61.26, 27.4)
  line L12 (-54.26, 2.6355) -> (-54.26, 20.4)
extrude "Extrude19'" add sketch "Sketch12" along normal mid plane 12.35 contours L0 A0 L1 L2 L3 L4 | A0 bodies 6 in component "Lid"
extrude "Extrude21" add sketch "Sketch12" along normal mid plane 3.2 contours L0 A0 L4 L6 L8 L9 L10 L11 L12 bodies 6 in component "Lid"
ref_plane "WorkPlane9" through (0, 0, 57.5) normal (0, 0, 1) x (1, 0, 0) in component "Lid"
sketch "Sketch13" plane through (0, 0, 57.5) normal (0, 0, 1) x (1, 0, 0) in component "Lid"
  line L0 (-60.2642, 29.9958) -> (-52.4, 22.1317)
  line L1 (-52.4, 25) -> (-54.26, 29.4)
  line L2 (-52.4, 25) -> (-52.4, 3.4059)
  line L3 (-54.26, 32.4) -> (-54.26, 29.4)
  circle A0 centre (-57.86, 32.4) radius 3.4
  circle A1 centre (-57.86, 32.4) radius 1.7
  line L4 (-54.26, 32.4) -> (-54.46, 32.4)
  line L5 (-61.26, 27.4) -> (-61.26, 3.0735)
  line L6 (-61.26, 27.4) -> (-61.26, 32.4)
  line L7 (-58.1865, 0) -> (-61.26, 3.0735)
  line L8 (-58.1865, 0) -> (-48, 0)
  line L9 (-48.9941, 0) -> (-52.4, 3.4059)
  line L10 (-51.6245, 0) -> (-54.26, 2.6355)
  line L11 (-54.26, 20.4) -> (-61.26, 27.4)
  line L12 (-54.26, 2.6355) -> (-54.26, 20.4)
extrude "Extrude20'" add sketch "Sketch13" along normal mid plane 12.35 contours L0 L1 L2 L3 A0 L4 | A0 bodies 6 in component "Lid"
extrude "Extrude22" add sketch "Sketch13" along normal mid plane 3.2 contours L0 L2 A0 L6 L8 L9 L10 L11 L12 bodies 6 in component "Lid"
fillet "Fillet2'" radius 1 34 edges at (52.4, 3.4059, 72.5) (50.2326, 3.4059, 80.2326) (38.5, 3.4059, 82.4) (54.26, 2.6355, 68.4) (54.26, 15.4, 68.4) (54.26, 15.4, 46.6) (54.26, 2.6355, 46.6) (52.4, 3.4059, 57.5) (52.4, 3.4059, 0) (54.26, 2.6355, -46.6) (54.26, 15.4, -46.6) (52.4, 3.4059, -57.5) (54.26, 2.6355, -68.4) (54.26, 15.4, -68.4) (38.5, 3.4059, -82.4) (50.2326, 3.4059, -80.2326) (52.4, 3.4059, -72.5) (29.5, 2.6355, -84.26) (0, 3.4059, -82.4) (-29.5, 2.6355, -84.26) (-52.4, 3.4059, -67.05) (-50.2326, 3.4059, -80.2326) (-38.5, 3.4059, -82.4) (-54.26, 2.6355, -57.5) (-54.26, 20.4, -57.5) (-52.4, 3.4059, 0) (-54.26, 2.6355, 57.5) (-54.26, 20.4, 57.5) (-38.5, 3.4059, 82.4) (-50.2326, 3.4059, 80.2326) (-52.4, 3.4059, 67.05) (0, 3.4059, 82.4) (-29.5, 2.6355, 84.26) (29.5, 2.6355, 84.26) 1 faces at (-16.3314, 0, -15) on bodies 6 in component "Lid"
fillet "Fillet3'" radius 3 6 edges at (-61.26, 27.4, -57.5) (-61.26, 27.4, 57.5) (61.26, 22.4, 68.4) (61.26, 22.4, 46.6) (61.26, 22.4, -46.6) (61.26, 22.4, -68.4) on bodies 6 in component "Lid"
copy_body "Body->Comp1'" bodies 6 removing the originals makes body 7 in component "Box Lid"
sketch "Sketch1 (3)" plane through (0, 0, 30.4) normal (0, 0, 1) x (-1, 0, 0) in component "Seal"
extrude "Extrude1''" add 1 faces at (-52.43, 30.4, -25) faces seen with x (0, -1, 0) y (0, 0, 1) z (-1, 0, 0) at (0, 0, 0) along direction (0, 0, 1) blind 1.4 separate body on bodies 2 makes body 8 in component "Seal"
mirror "Mirror2" about plane through (324.9667, 84.4068, 66.6) normal (0, 0, 1) of bodies 4 makes body 9 in component "Box Latch"
sketch "Sketch1 (4)" plane through (0, 0, 2.4) normal (0, 0, 1) x (-1, 0, 0)
  arc A0 (78, -70.72) -> (75, -67.72) centre (75, -70.72) ccw
  line L0 (75, -67.72) -> (-75, -67.72)
  arc A1 (-75, -67.72) -> (-78, -70.72) centre (-75, -70.72) ccw
  line L1 (-78, -70.72) -> (-78, -160.72)
  arc A2 (-78, -160.72) -> (-75, -163.72) centre (-75, -160.72) ccw
  line L2 (-75, -163.72) -> (75, -163.72)
  arc A3 (75, -163.72) -> (78, -160.72) centre (75, -160.72) ccw
  line L3 (78, -160.72) -> (78, -70.72)
sketch "Sketch2 (3)" plane through (0, 0, 2.4) normal (0, 0, 1) x (1, 0, 0)